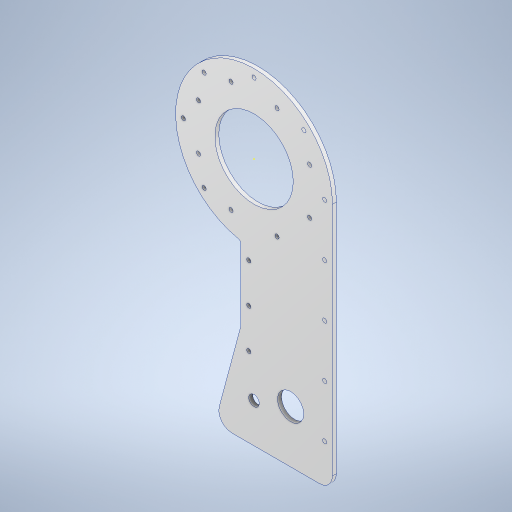
# Autodesk Inventor part: RP_Thigh-cover
Saved by Autodesk Inventor 2024.3 (Build 283343000, 343)
## iProperties
Created: 2024-10-20
Part Number: RP_Thigh-cover
Material: アルミニウム 6061
Document SubType Name: Modeling
Designer: 佐藤智貴
Density: 2.7 g/cm^3
Appearance: アルミニウム - フラット
Mass: 144.192 g
Surface Area: 389.937 cm^2
Volume: 53.4046 cm^3
Author: 佐藤智貴
Autodesk Inventor part; units mm, degrees
ref_plane "YZ Plane" through (0, 0, 0) normal (1, 0, 0) x (0, 1, 0)
ref_plane "XZ Plane" through (0, 0, 0) normal (0, 1, 0) x (-1, 0, 0)
ref_plane "XY Plane" through (0, 0, 0) normal (0, 0, 1) x (1, 0, 0)
sketch "スケッチ1" plane through (0, 0, 0) normal (0, 0, 1) x (1, 0, 0)
  circle A0 centre (0, 0) radius 60
  dimension "d0" = 120
  constraints: 1 centre point, 1 coincident
  measures "d0" diameter of A0
extrude "押し出し1" add sketch "スケッチ1" along normal blind 3
sketch "スケッチ2" plane through (0, 0, 3) normal (0, 0, 1) x (1, 0, 0)
  circle A0 centre (0, 0) radius 46
  line L0 (0, 0) -> (0, 59.211)
  line L1 (0, 0) -> (-21.8609, 52.777)
  line L2 (0, 0) -> (27.8226, 47.8581)
  point P0 (-17.6034, 42.4985)
  point P1 (-42.4985, 17.6034)
  point P2 (-42.4985, -17.6034)
  point P3 (-17.6034, -42.4985)
  point P4 (17.6034, -42.4985)
  point P5 (42.4985, -17.6034)
  point P6 (42.4985, 17.6034)
  point P7 (17.6034, 42.4985)
  dimension "d4" = 92
  dimension "d5" = 22.5
  dimension "d8" = 360
  constraints: 6 end point, 1 coincident, 1 point on line, 1 vertical, 12 other
  measures "d5" angle of L1 L0
hole "穴1" at (-17.6034, 42.4985, 3) at (-42.4985, 17.6034, 3) at (-42.4985, -17.6034, 3) at (-17.6034, -42.4985, 3) at (17.6034, -42.4985, 3) at (42.4985, -17.6034, 3) at (42.4985, 17.6034, 3) at (17.6034, 42.4985, 3) direction (0, 0, -1) diameter 3.2 end through all
sketch "スケッチ4" plane through (0, 0, 0) normal (0, 0, -1) x (-1, 0, 0)
  line L0 (0, 0) -> (0, -80.557)
  circle A0 centre (0, 0) radius 60 projected
  line L1 (-60, 0) -> (-60, -190)
  line L2 (60, 0) -> (60, -190)
  line L3 (-60, -190) -> (60, -190)
  line L4 (-60, 0) -> (-43.3772, -190)
  line L5 (10.9847, -144.6101) -> (60, -190)
  line L6 (18.2202, -151.3104) -> (-10.1159, -125.0702)
  line L7 (10, -105.557) -> (10, -25)
  circle A1 centre (0, 0) radius 7 projected
  line L8 (10, -177.6776) -> (0, -177.6776)
  line L9 (0, -177.6776) -> (0, -62.3224)
  line L10 (10, -62.3224) -> (10, -177.6776)
  circle A2 centre (0, -160) radius 4
  circle A3 centre (0, -160) radius 15
  line L11 (27.6237, -152.2466) -> (-9.3418, -192.1645)
  line L12 (15, -160) -> (15, -138.6677)
  line L13 (30, -190) -> (10, -115.4165)
  point P0 (60, 0)
  point P1 (-59.0885, -10.4189)
  point P2 (-60, -25)
  point P3 (60, -25)
  point P4 (10, -59.1608)
  point P5 (10, -143.6982)
  point P6 (0, -134.4378)
  point P7 (0, -60)
  point P8 (0, -60)
  point P9 (10, -120)
  point P10 (10, -171.1803)
  point P11 (11.0058, -170.1918)
  point P12 (10, -171.2779)
  point P13 (21.6159, -158.7342)
  point P14 (-7.3373, -190)
  dimension "d362" = 30
  dimension "d21" = 60
  dimension "d23" = 120
  dimension "d24" = 190
  dimension "d25" = 190
  dimension "d56" = 0
  dimension "d90" = 85
  dimension "d307" = 10
  dimension "d359" = 160
  dimension "d361" = 8
  dimension "d379" = 30
  dimension "d380" = 0
  dimension "d381" = 70
  constraints: 28 end point, 7 point on line, 3 perpendicular, 3 vertical, 1 centre point, 1 horizontal, 1 midpoint, 1 parallel, 7 other
  measures "d21" distance from line of L1 L0.start
  measures "d23" distance between parallel lines of L2 L1
  measures "d24" distance of L2.start L2.end
  measures "d25" distance of L1.start L1.end
  measures "d56" angle of L2 L0
  measures "d90" angle of L3 L4
  measures "d307" distance between parallel lines of L7 L0
  measures "d359" distance of A2.centre point (0, 0)
  measures "d361" diameter of A2
  measures "d379" distance from line of L2 L13.start
  measures "d380" distance between parallel lines of L7 L10
  measures "d381" distance from line of L3 point (10, -120)
extrude "押し出し3" add sketch "スケッチ4" against normal blind 3 contours L0 A0 L7 L10 L6 L9 | L0 L9 A3 L8 L11 L3 L4 A0 | L6 L10 A3 L9 | L4 L3 L1 A0 | L10 L13 L5 L6 | L6 L5 L12 A3 L10 | A3 L10 L9 A2 | L9 A2 A3 | A3 L10 | A3 L10 L11 L8 L9 | L11 L8 L10 L13 L3 | L5 L13 L11 A3 L12 | A3 L11 L10 | L11 L10 L8
sketch "スケッチ17" plane through (0, 0, 3) normal (0, 0, 1) x (1, 0, 0)
  circle A0 centre (0, 0) radius 30
  dimension "d159" = 60
  constraints: 1 centre point, 1 coincident
  measures "d159" diameter of A0
extrude "押し出し10" cut sketch "スケッチ17" against normal blind 10
sketch "スケッチ20" plane through (0, 0, 3) normal (0, 0, 1) x (1, 0, 0)
  line L0 (-30, -190) -> (60, -190) projected
  circle A0 centre (0, 0) radius 30 projected
  line L1 (60, -190) -> (60, 0) projected
  point P0 (0, -160)
  point P1 (15, -190)
  point P2 (-60, -190)
  point P3 (7.3373, -190)
  dimension "d205" = 160
  dimension "d223" = 60
  dimension "d246" = 60
  constraints: 1 midpoint
  measures "d205" distance of point (0, -160) A0.centre
  measures "d223" distance from line of L1 point (0, -160)
  measures "d246" distance from line of point (0, 0) L1
hole "穴8" at (0, -160, 3) direction (0, 0, -1) diameter 8.1 end through all
fillet "フィレット4" radius 10 3 edges at (60, -190, 1.5) (-10, -115.4165, 1.5) (-30, -190, 1.5)
sketch "スケッチ28" plane through (0, 0, 3) normal (0, 0, 1) x (1, 0, 0)
  circle A0 centre (0, 0) radius 60
  circle A1 centre (0, 0) radius 54
  point P0 (0, 54)
  point P1 (-38.1838, 38.1838)
  point P2 (-54, 0)
  point P3 (-38.1838, -38.1838)
  point P4 (0, -54)
  point P5 (38.1838, -38.1838)
  point P6 (54, 0)
  point P7 (38.1838, 38.1838)
  dimension "d309" = 108
  dimension "d308" = 120
  dimension "d312" = 360
  constraints: 1 centre point, 1 coincident, 1 vertical alignment, 11 other
  measures "d308" diameter of A0
hole "穴13" at (-38.1838, -38.1838, 3) at (-54, 0, 3) at (-38.1838, 38.1838, 3) at (0, 54, 3) at (38.1838, 38.1838, 3) at (54, 0, 3) direction (0, 0, -1) diameter 3.2 end through all
sketch "スケッチ29" plane through (0, 0, 3) normal (0, 0, 1) x (1, 0, 0)
  arc A0 (60, 0) -> (-10, -59.1608) centre (0, 0) ccw projected
  line L0 (-10, -59.1608) -> (0, -59.1608)
  line L1 (0, -59.1608) -> (0, -130)
  line L2 (0, -130) -> (-10, -130)
  line L3 (-10, -130) -> (-10, -59.1608)
  line L4 (60, 0) -> (60, -180) projected
  line L5 (60, -130) -> (50, -130)
  line L6 (50, -130) -> (50, 10.2883)
  line L7 (50, 10.2883) -> (60, 10.2883)
  line L8 (60, 10.2883) -> (60, -130)
  line L9 (-30, -190) -> (50, -190) projected
  circle A1 centre (54, 0) radius 1.6 projected
  line L10 (-10, -59.1608) -> (-10, -115.4165) projected
  point P0 (-35.8579, -190)
  point P1 (54, -40)
  point P2 (-5, -59.1608)
  point P3 (-4, -69.1608)
  point P4 (54, -80)
  point P5 (54, -120)
  point P6 (54, -160)
  point P7 (55, -130)
  point P8 (-5, -130)
  point P9 (-4, -129.1608)
  point P10 (54, -200)
  point P11 (-10, -140)
  point P12 (40, -210)
  point P13 (-40, -210)
  point P14 (-4, -99.1608)
  point P15 (7.3373, -190)
  point P16 (11.7061, -190)
  dimension "d321" = 60
  dimension "d322" = 10
  dimension "d323" = 10
  dimension "d324" = 40
  dimension "d325" = 6
  dimension "d339" = 40
  dimension "d340" = 40
  dimension "d341" = 40
  dimension "d342" = 6
  dimension "d352" = 4
  dimension "d356" = 40
  dimension "d357" = 6
  dimension "d358" = 6
  dimension "d364" = 10
  dimension "d366" = 4
  dimension "d367" = 30
  dimension "d368" = 30
  constraints: 16 end point, 4 parallel, 3 midpoint, 2 horizontal, 2 perpendicular, 2 point on line, 1 other
  measures "d322" distance between parallel lines of L3 L1
  measures "d323" distance between parallel lines of L4 L6
  measures "d324" distance of A1.centre point (54, -40)
  measures "d325" distance from line of L4 point (54, -40)
  measures "d339" distance of point (54, -160) point (54, -120)
  measures "d340" distance of point (54, -40) point (54, -80)
  measures "d341" distance of point (54, -120) point (54, -80)
  measures "d342" distance from line of L4 point (54, -160)
  measures "d352" distance from line of L1 point (-4, -69.161)
  measures "d356" distance of point (54, -160) point (54, -200)
  measures "d357" distance from line of L4 point (54, -200)
  measures "d358" distance from line of L10 point (-4, -129.161)
  measures "d364" distance from line of point (-4, -69.161) L0
  measures "d366" distance from line of L1 point (-4, -99.161)
  measures "d367" distance of point (-4, -69.161) point (-4, -99.161)
  measures "d368" distance of point (-4, -129.161) point (-4, -99.161)
hole "穴14" at (54, -80, 3) at (54, -200, 3) at (54, -160, 3) at (54, -120, 3) at (54, -40, 3) at (-4, -69.1608, 3) at (-4, -99.1608, 3) at (-4, -129.1608, 3) direction (0, 0, -1) diameter 3.2 end through all
fillet "フィレット11" radius 2.5 1 edges at (-10, -59.1608, 1.5)
sketch "スケッチ30" plane through (0, 0, 3) normal (0, 0, 1) x (1, 0, 0)
  point P0 (0, 0)
sketch "スケッチ32" plane through (0, 0, 3) normal (0, 0, 1) x (1, 0, 0)
  circle A0 centre (28, -150) radius 10
  line L0 (60, -180) -> (60, 0) projected
  point P0 (0, 0)
  dimension "d382" = 20
  dimension "d383" = 150
  dimension "d384" = 32
  constraints: 1 centre point
  measures "d382" diameter of A0
  measures "d383" vertical distance of point (0, 0) A0.centre
  measures "d384" distance from line of L0 A0.centre
extrude "押し出し16" cut sketch "スケッチ32" against normal blind 10
equation "\"d25\" = d24"
equation "\"d90\" = d89"
equation "\"d89\" = 85deg"
